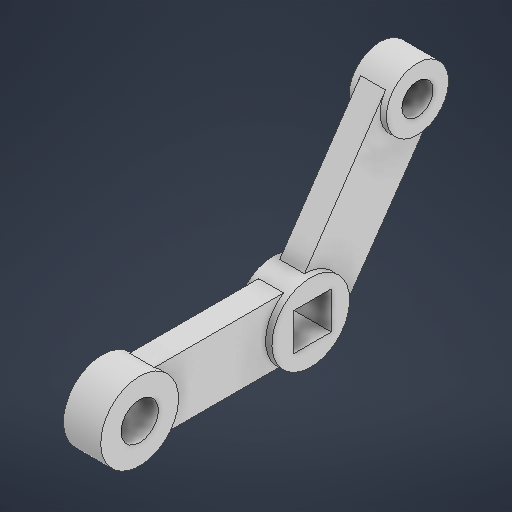
# Autodesk Inventor part: Tipo1
Saved by Autodesk Inventor 2026 (Build 300175050, 175E)
## iProperties
Created: 2026-04-09
Part Number: Tipo1
Material: Generic
Document SubType Name: Modeling
Designer: Administrator
Density: 1 g/cm^3
Appearance: Default
Author: Administrator
Autodesk Inventor part; units mm, degrees
ref_plane "YZ Plane" through (0, 0, 0) normal (1, 0, 0) x (0, 1, 0)
ref_plane "XZ Plane" through (0, 0, 0) normal (0, 1, 0) x (-1, 0, 0)
ref_plane "XY Plane" through (0, 0, 0) normal (0, 0, 1) x (1, 0, 0)
sketch "Sketch4" plane through (0, 0, 0) normal (1, 0, 0) x (0, 1, 0)
  line L0 (0, 0) -> (0, -55)
  line L1 (0, -55) -> (45, -89.2919)
  circle A0 centre (0, 0) radius 12.5
  circle A1 centre (0, 0) radius 6
  circle A2 centre (0, -55) radius 12.5
  circle A3 centre (45, -89.2919) radius 10
  circle A4 centre (45, -89.2919) radius 5
  line L2 (8.7921, -8.8853) -> (8.7921, -46.1147)
  line L3 (-11.2079, -5.5348) -> (-11.2079, -49.4652)
  line L4 (-6, -65.9659) -> (37.4603, -95.861)
  line L5 (12.4075, -56.5181) -> (50.3971, -80.8734)
  point P0 (0, -50.7919)
  dimension "d15" = 10
  dimension "d16" = 20
  dimension "d17" = 25
  dimension "d18" = 12
  dimension "d19" = 25
  dimension "d20" = 20
  dimension "d24" = 45
  dimension "d29" = 55
  constraints: 12 end point, 8 point on circle, 5 centre point, 5 coincident, 3 vertical, 1 tangent
  measures "d15" diameter of A4
  measures "d16" diameter of A3
  measures "d17" diameter of A2
  measures "d18" diameter of A1
  measures "d19" diameter of A0
  measures "d20" distance between parallel lines of L3 L2
  measures "d24" horizontal distance of L0.end L1.end
  measures "d29" distance of L0.start L0.end
extrude "Extrusion2" add sketch "Sketch4" along normal mid plane 12 contours A0 | A2 L1 L0 | L0 L1 A2 | A3 | A4
sketch "Sketch5" plane through (6, 0, 0) normal (1, 0, 0) x (0, 0, -1)
  circle A0 centre (0, 0) radius 12.5 projected
  line L0 (6.7288, 10.5344) -> (48.2712, 10.5344)
  circle A1 centre (55, 0) radius 12.5 projected
  line L1 (55, 12.5) -> (81.0326, 50.6377)
  circle A2 centre (89.2919, 45) radius 10 projected
  line L2 (65.8713, -6.1697) -> (97.565, 39.3813)
  line L3 (8.1641, -9.4656) -> (46.8359, -9.4656)
  point P0 (97.5005, 39.2886)
  dimension "d34" = 20
  constraints: 8 end point, 6 point on circle, 2 horizontal, 4 other
  measures "d34" distance between parallel lines of L3 L0
extrude "Extrusion3" add sketch "Sketch5" against normal blind 12 separate body contours A0 L0 A1 L3 | L1 A2 L2 A1
sketch "Sketch7" plane through (6, 45, -89.2919) normal (1, 0, 0) x (0, 0, -1)
  line L0 (-39.6827, -39) -> (-27.6827, -39)
  line L1 (-27.6827, -39) -> (-27.6827, -51)
  line L2 (-27.6827, -51) -> (-39.6827, -51)
  line L3 (-39.6827, -51) -> (-39.6827, -39)
  line L4 (-89.2919, -45) -> (-34.2919, -45)
  point P0 (-33.6827, -39)
  point P1 (-27.6827, -45)
  dimension "d42" = 55
  dimension "d43" = 12
  dimension "d44" = 12
  dimension "d45" = 6
  constraints: 10 end point, 2 horizontal, 2 midpoint, 2 parallel, 1 perpendicular
  measures "d42" distance of L4.start L4.end
  measures "d43" distance from line of L2 point (-33.683, -39)
  measures "d44" distance from line of L3 point (-27.683, -45)
  measures "d45" distance from line of L4.end L2
extrude "Extrusion5" cut sketch "Sketch7" against normal blind 12 bodies 1
sketch "Sketch9" plane through (6, 45, -89.2919) normal (1, 0, 0) x (0, 0, -1)
  circle A0 centre (0, 0) radius 5
  point P0 (-89.2919, -45)
  dimension "d48" = 10
  constraints: 1 centre point
  measures "d48" diameter of A0
extrude "Extrusion6" cut sketch "Sketch9" against normal blind 12 bodies 1
sketch "Sketch11" plane through (6, 0, 0) normal (1, 0, 0) x (0, 0, -1)
  line L0 (6.7288, 10.5344) -> (48.2712, 10.5344) projected
  arc A0 (48.2712, 10.5344) -> (46.8359, -9.4656) centre (55, 0) ccw projected
  line L1 (6.7288, 10.5344) -> (48.2712, 10.5344)
  arc A1 (8.1641, -9.4656) -> (6.7288, 10.5344) centre (0, 0) ccw projected
  line L2 (8.1641, -9.4656) -> (46.8359, -9.4656) projected
  line L3 (8.1641, -9.4656) -> (46.8359, -9.4656)
  line L4 (0, 0) -> (55, 0)
  arc A2 (8.1641, -9.4656) -> (6.7288, 10.5344) centre (0, 0) ccw
  arc A3 (48.2712, 10.5344) -> (46.8359, -9.4656) centre (55, 0) ccw
  constraints: 6 end point, 4 point on circle, 3 horizontal, 2 centre point, 2 concentric
extrude "Extrusion7" cut sketch "Sketch11" against normal blind 2 bodies 2
sketch "Sketch12" plane through (6, 0, 0) normal (1, 0, 0) x (0, 0, -1)
  circle A0 centre (55, 0) radius 12.5 projected
  line L0 (97.5005, 39.2886) -> (65.8713, -6.1697) projected
  line L1 (65.8713, -6.1697) -> (97.5005, 39.2886)
  arc A1 (65.8713, -6.1697) -> (55, 12.5) centre (55, 0) ccw
  line L2 (55, 12.5) -> (81.0326, 50.6377) projected
  line L3 (55, 12.5) -> (81.0326, 50.6377)
  arc A2 (81.0326, 50.6377) -> (97.5005, 39.2886) centre (89.2919, 45) ccw
  point P0 (0, 0)
  constraints: 6 point on circle, 4 end point, 2 centre point, 2 collinear, 2 tangent, 1 concentric
extrude "Extrusion8" cut sketch "Sketch12" against normal blind 2 contours A0 L2 A2 L0 bodies 2
sketch "Sketch13" plane through (-6, 0, 0) normal (-1, 0, 0) x (0, 0, 1)
  circle A0 centre (-55, 0) radius 12.5 projected
  line L0 (-48.2846, 10.5429) -> (-6.6455, 10.5429)
  circle A1 centre (0, 0) radius 12.5 projected
  line L1 (-46.8359, -9.4656) -> (-8.1641, -9.4656) projected
  line L2 (-8.1641, -9.4656) -> (-46.8359, -9.4656)
  arc A2 (-46.8359, -9.4656) -> (-48.2846, 10.5429) centre (-55, 0) ccw
  arc A3 (-6.6455, 10.5429) -> (-8.1641, -9.4656) centre (-0.0437, -0.02) ccw
  point P0 (-12.5, 0)
  point P1 (-6.7154, 10.5429)
  constraints: 6 point on circle, 4 end point, 2 centre point, 1 collinear, 1 concentric, 1 horizontal
extrude "Extrusion9" cut sketch "Sketch13" against normal blind 2 contours A0 L0 A1 A3 L1 bodies 2
sketch "Sketch14" plane through (-6, 0, 0) normal (-1, 0, 0) x (0, 0, 1)
  circle A0 centre (-89.2919, 45) radius 10 projected
  circle A1 centre (-55, 0) radius 12.5 projected
  line L0 (-97.5005, 39.2886) -> (-65.8713, -6.1697) projected
  line L1 (-97.5005, 39.2886) -> (-65.8713, -6.1697)
  arc A2 (-97.5005, 39.2886) -> (-81.0326, 50.6377) centre (-89.2919, 45) ccw
  arc A3 (-55, 12.5) -> (-65.8713, -6.1697) centre (-55, 0) ccw
  line L2 (-55, 12.5) -> (-81.0326, 50.6377) projected
  line L3 (-81.0326, 50.6377) -> (-55, 12.5)
  point P0 (0, 0)
  constraints: 6 point on circle, 4 end point, 3 concentric, 2 centre point, 1 collinear, 1 tangent
extrude "Extrusion10" cut sketch "Sketch14" against normal blind 2 contours A0 L2 A1 L0 bodies 2
body "Solid2"
body "Solid3"
